Autodesk Inventor part; units mm, degrees
(part 2 of 2)
sketch "Sketch23" plane through (0, 0, 0) normal (0, 0, -1) x (-1, 0, 0)
  line L0 (124.7957, 172.4284) -> (124.7957, 166.0784) projected
  line L1 (124.7957, 166.0784) -> (73.9957, 166.0784) projected
  line L2 (73.9957, 166.0784) -> (73.9957, 172.4284) projected
  line L3 (73.9957, 172.4284) -> (23.1957, 172.4284) projected
  line L4 (23.1957, 172.4284) -> (23.1957, 166.0784) projected
  line L5 (23.1957, 166.0784) -> (-27.6043, 166.0784) projected
  line L6 (-27.6043, 166.0784) -> (-27.6043, 172.4284) projected
  line L7 (-27.6043, 172.4284) -> (-78.4043, 172.4284) projected
  line L8 (-78.4043, 172.4284) -> (-78.4043, 166.0784) projected
  line L9 (-78.4043, 166.0784) -> (-129.2043, 166.0784) projected
  line L10 (-129.2043, 166.0784) -> (-129.2043, 172.4284) projected
  line L11 (-129.2043, 172.4284) -> (-180.0043, 172.4284) projected
  line L12 (-180.0043, 172.4284) -> (-180.0043, 166.0784) projected
  line L13 (-180.0043, 166.0784) -> (-230.8043, 166.0784) projected
  line L14 (-230.8043, 166.0784) -> (-230.8043, 172.4284) projected
  line L15 (-230.8043, 172.4284) -> (-281.6043, 172.4284) projected
  line L16 (-281.6043, 172.4284) -> (-281.6043, 166.0784) projected
  line L17 (-281.6043, 166.0784) -> (-332.4043, 166.0784) projected
  line L18 (-332.4043, 166.0784) -> (-332.4043, 172.4284) projected
  line L19 (-332.4043, 172.4284) -> (-351.4543, 172.4284) projected
  line L20 (-351.4543, 172.4284) -> (-351.4543, 121.6284) projected
  line L21 (-351.4543, 121.6284) -> (-345.1043, 121.6284) projected
  line L22 (-345.1043, 121.6284) -> (-345.1043, 70.8284) projected
  line L23 (-345.1043, 70.8284) -> (-351.4543, 70.8284) projected
  line L24 (-351.4543, 70.8284) -> (-351.4543, 20.0284) projected
  line L25 (-351.4543, 20.0284) -> (-345.1043, 20.0284) projected
  line L26 (-345.1043, 20.0284) -> (-345.1043, -30.7716) projected
  line L27 (-345.1043, -30.7716) -> (-351.4543, -30.7716) projected
  line L28 (-351.4543, -30.7716) -> (-351.4543, -81.5716) projected
  line L29 (-351.4543, -81.5716) -> (-345.1043, -81.5716) projected
  line L30 (-345.1043, -81.5716) -> (-345.1043, -132.3716) projected
  line L31 (-345.1043, -132.3716) -> (-351.4543, -132.3716) projected
  line L32 (-351.4543, -132.3716) -> (-351.4543, -183.1716) projected
  line L33 (-351.4543, -183.1716) -> (-345.1043, -183.1716) projected
  line L34 (-345.1043, -183.1716) -> (-345.1043, -233.9716) projected
  line L35 (-345.1043, -233.9716) -> (-351.4543, -233.9716) projected
  line L36 (-351.4543, -233.9716) -> (-351.4543, -284.7716) projected
  line L37 (-351.4543, -284.7716) -> (-345.1043, -284.7716) projected
  line L38 (-345.1043, -284.7716) -> (-345.1043, -335.5716) projected
  line L39 (-345.1043, -335.5716) -> (-351.4543, -335.5716) projected
  line L40 (-351.4543, -335.5716) -> (-351.4543, -386.3716) projected
  line L41 (-351.4543, -386.3716) -> (-345.1043, -386.3716) projected
  line L42 (-345.1043, -386.3716) -> (-345.1043, -437.1716) projected
  line L43 (-345.1043, -437.1716) -> (-351.4543, -437.1716) projected
  line L44 (-351.4543, -437.1716) -> (-351.4543, -487.9716) projected
  line L45 (-351.4543, -487.9716) -> (-345.1043, -487.9716) projected
  line L46 (-345.1043, -487.9716) -> (-345.1043, -538.7716) projected
  line L47 (-345.1043, -538.7716) -> (-351.4543, -538.7716) projected
  line L48 (-351.4543, -538.7716) -> (-351.4543, -589.5716) projected
  line L49 (-351.4543, -589.5716) -> (-345.1043, -589.5716) projected
  line L50 (-345.1043, -589.5716) -> (-345.1043, -640.3716) projected
  line L51 (-345.1043, -640.3716) -> (-351.4543, -640.3716) projected
  line L52 (-351.4543, -640.3716) -> (-351.4543, -716.5716) projected
  line L53 (-351.4543, -716.5716) -> (-332.4043, -716.5716) projected
  line L54 (-332.4043, -716.5716) -> (-332.4043, -710.2216) projected
  line L55 (-332.4043, -710.2216) -> (-281.6043, -710.2216) projected
  line L56 (-281.6043, -710.2216) -> (-281.6043, -716.5716) projected
  line L57 (-281.6043, -716.5716) -> (-230.8043, -716.5716) projected
  line L58 (-230.8043, -716.5716) -> (-230.8043, -710.2216) projected
  line L59 (-230.8043, -710.2216) -> (-180.0043, -710.2216) projected
  line L60 (-180.0043, -710.2216) -> (-180.0043, -716.5716) projected
  line L61 (-180.0043, -716.5716) -> (-129.2043, -716.5716) projected
  line L62 (-129.2043, -716.5716) -> (-129.2043, -710.2216) projected
  line L63 (-129.2043, -710.2216) -> (-78.4043, -710.2216) projected
  line L64 (-78.4043, -710.2216) -> (-78.4043, -716.5716) projected
  line L65 (-78.4043, -716.5716) -> (-27.6043, -716.5716) projected
  line L66 (-27.6043, -716.5716) -> (-27.6043, -710.2216) projected
  line L67 (-27.6043, -710.2216) -> (23.1957, -710.2216) projected
  line L68 (23.1957, -710.2216) -> (23.1957, -716.5716) projected
  line L69 (23.1957, -716.5716) -> (73.9957, -716.5716) projected
  line L70 (73.9957, -716.5716) -> (73.9957, -710.2216) projected
  line L71 (73.9957, -710.2216) -> (124.7957, -710.2216) projected
  line L72 (124.7957, -710.2216) -> (124.7957, -716.5716) projected
  line L73 (124.7957, -716.5716) -> (143.8457, -716.5716) projected
  line L74 (143.8457, -716.5716) -> (143.8457, -640.3716) projected
  line L75 (143.8457, -640.3716) -> (137.4957, -640.3716) projected
  line L76 (137.4957, -640.3716) -> (137.4957, -589.5716) projected
  line L77 (137.4957, -589.5716) -> (143.8457, -589.5716) projected
  line L78 (143.8457, -589.5716) -> (143.8457, -538.7716) projected
  line L79 (143.8457, -538.7716) -> (137.4957, -538.7716) projected
  line L80 (137.4957, -538.7716) -> (137.4957, -487.9716) projected
  line L81 (137.4957, -487.9716) -> (143.8457, -487.9716) projected
  line L82 (143.8457, -487.9716) -> (143.8457, -437.1716) projected
  line L83 (143.8457, -437.1716) -> (137.4957, -437.1716) projected
  line L84 (137.4957, -437.1716) -> (137.4957, -386.3716) projected
  line L85 (137.4957, -386.3716) -> (143.8457, -386.3716) projected
  line L86 (143.8457, -386.3716) -> (143.8457, -335.5716) projected
  line L87 (143.8457, -335.5716) -> (137.4957, -335.5716) projected
  line L88 (137.4957, -335.5716) -> (137.4957, -284.7716) projected
  line L89 (137.4957, -284.7716) -> (143.8457, -284.7716) projected
  line L90 (143.8457, -284.7716) -> (143.8457, -233.9716) projected
  line L91 (143.8457, -233.9716) -> (137.4957, -233.9716) projected
  line L92 (137.4957, -233.9716) -> (137.4957, -183.1716) projected
  line L93 (137.4957, -183.1716) -> (143.8457, -183.1716) projected
  line L94 (143.8457, -183.1716) -> (143.8457, -132.3716) projected
  line L95 (143.8457, -132.3716) -> (137.4957, -132.3716) projected
  line L96 (137.4957, -132.3716) -> (137.4957, -81.5716) projected
  line L97 (137.4957, -81.5716) -> (143.8457, -81.5716) projected
  line L98 (143.8457, -81.5716) -> (143.8457, -30.7716) projected
  line L99 (143.8457, -30.7716) -> (137.4957, -30.7716) projected
  line L100 (137.4957, -30.7716) -> (137.4957, 20.0284) projected
  line L101 (137.4957, 20.0284) -> (143.8457, 20.0284) projected
  line L102 (143.8457, 20.0284) -> (143.8457, 70.8284) projected
  line L103 (143.8457, 70.8284) -> (137.4957, 70.8284) projected
  line L104 (137.4957, 70.8284) -> (137.4957, 121.6284) projected
  line L105 (137.4957, 121.6284) -> (143.8457, 121.6284) projected
  line L106 (143.8457, 121.6284) -> (143.8457, 172.4284) projected
  line L107 (143.8457, 172.4284) -> (124.7957, 172.4284) projected
  line L108 (-351.4543, 172.4284) -> (143.8457, 172.4284)
  line L109 (143.8457, 172.4284) -> (143.8457, -716.5716)
  line L110 (143.8457, -716.5716) -> (-351.4543, -716.5716)
  line L111 (-351.4543, -716.5716) -> (-351.4543, 172.4284)
  line L112 (124.7957, -699.4992) -> (-323.907, -699.4992)
  line L113 (-323.907, -699.4992) -> (-323.907, 137.5099)
  line L114 (-323.907, 137.5099) -> (124.7957, 137.5099)
  line L115 (124.7957, 137.5099) -> (124.7957, -699.4992)
  point P0 (0, 0)
  constraints: 16 end point, 4 parallel, 2 horizontal, 2 perpendicular
extrude "Extrusion23" add sketch "Sketch23" against normal blind 6.35 contours L107 L106 L105 L104 L103 L102 L101 L100 L99 L98 L97 L96 L95 L94 L93 L92 L91 L90 L89 L88 L87 L86 L85 L84 L83 L82 L81 L80 L79 L78 L77 L76 L75 L74 L73 L72 L71 L70 L69 L68 L67 L66 L65 L64 L63 L62 L61 L60 L59 L58 L57 L56 L55 L54 L53 L52 L51 L50 L49 L48 L47 L46 L45 L44 L43 L42 L41 L40 L39 L38 L37 L36 L35 L34 L33 L32 L31 L30 L29 L28 L27 L26 L25 L24 L23 L22 L21 L20 L19 L18 L17 L16 L15 L14 L13 L12 L11 L10 L9 L8 L7 L6 L5 L4 L3 L2 L1 L0 | L0 L1 L2 L108 | L109 L103 L104 L105 | L4 L5 L6 L108 | L109 L99 L100 L101 | L8 L9 L10 L108 | L109 L95 L96 L97 | L12 L13 L14 L108 | L109 L91 L92 L93 | L16 L17 L18 L108 | L109 L87 L88 L89 | L109 L83 L84 L85 | L109 L79 L80 L81 | L109 L75 L76 L77
sketch "Sketch24" plane through (0, 0, 0) normal (0, 0, -1) x (-1, 0, 0)
  line L0 (143.8457, 172.4284) -> (-351.4543, 172.4284) projected
  line L1 (-351.4543, 172.4284) -> (-351.4543, 121.6284) projected
  line L2 (-351.4543, 121.6284) -> (-345.1043, 121.6284) projected
  line L3 (-345.1043, 121.6284) -> (-345.1043, 70.8284) projected
  line L4 (-345.1043, 70.8284) -> (-351.4543, 70.8284) projected
  line L5 (-351.4543, 70.8284) -> (-351.4543, 20.0284) projected
  line L6 (-351.4543, 20.0284) -> (-345.1043, 20.0284) projected
  line L7 (-345.1043, 20.0284) -> (-345.1043, -30.7716) projected
  line L8 (-345.1043, -30.7716) -> (-351.4543, -30.7716) projected
  line L9 (-351.4543, -30.7716) -> (-351.4543, -81.5716) projected
  line L10 (-351.4543, -81.5716) -> (-345.1043, -81.5716) projected
  line L11 (-345.1043, -81.5716) -> (-345.1043, -132.3716) projected
  line L12 (-345.1043, -132.3716) -> (-351.4543, -132.3716) projected
  line L13 (-351.4543, -132.3716) -> (-351.4543, -183.1716) projected
  line L14 (-351.4543, -183.1716) -> (-345.1043, -183.1716) projected
  line L15 (-345.1043, -183.1716) -> (-345.1043, -233.9716) projected
  line L16 (-345.1043, -233.9716) -> (-351.4543, -233.9716) projected
  line L17 (-351.4543, -233.9716) -> (-351.4543, -284.7716) projected
  line L18 (-351.4543, -284.7716) -> (-345.1043, -284.7716) projected
  line L19 (-345.1043, -284.7716) -> (-345.1043, -335.5716) projected
  line L20 (-345.1043, -335.5716) -> (-351.4543, -335.5716) projected
  line L21 (-351.4543, -335.5716) -> (-351.4543, -386.3716) projected
  line L22 (-351.4543, -386.3716) -> (-345.1043, -386.3716) projected
  line L23 (-345.1043, -386.3716) -> (-345.1043, -437.1716) projected
  line L24 (-345.1043, -437.1716) -> (-351.4543, -437.1716) projected
  line L25 (-351.4543, -437.1716) -> (-351.4543, -487.9716) projected
  line L26 (-351.4543, -487.9716) -> (-345.1043, -487.9716) projected
  line L27 (-345.1043, -487.9716) -> (-345.1043, -538.7716) projected
  line L28 (-345.1043, -538.7716) -> (-351.4543, -538.7716) projected
  line L29 (-351.4543, -538.7716) -> (-351.4543, -589.5716) projected
  line L30 (-351.4543, -589.5716) -> (-345.1043, -589.5716) projected
  line L31 (-345.1043, -589.5716) -> (-345.1043, -640.3716) projected
  line L32 (-345.1043, -640.3716) -> (-351.4543, -640.3716) projected
  line L33 (-351.4543, -640.3716) -> (-351.4543, -716.5716) projected
  line L34 (-351.4543, -716.5716) -> (-332.4043, -716.5716) projected
  line L35 (-332.4043, -716.5716) -> (-332.4043, -710.2216) projected
  line L36 (-332.4043, -710.2216) -> (-281.6043, -710.2216) projected
  line L37 (-281.6043, -710.2216) -> (-281.6043, -716.5716) projected
  line L38 (-281.6043, -716.5716) -> (-230.8043, -716.5716) projected
  line L39 (-230.8043, -716.5716) -> (-230.8043, -710.2216) projected
  line L40 (-230.8043, -710.2216) -> (-180.0043, -710.2216) projected
  line L41 (-180.0043, -710.2216) -> (-180.0043, -716.5716) projected
  line L42 (-180.0043, -716.5716) -> (-129.2043, -716.5716) projected
  line L43 (-129.2043, -716.5716) -> (-129.2043, -710.2216) projected
  line L44 (-129.2043, -710.2216) -> (-78.4043, -710.2216) projected
  line L45 (-78.4043, -710.2216) -> (-78.4043, -716.5716) projected
  line L46 (-78.4043, -716.5716) -> (-27.6043, -716.5716) projected
  line L47 (-27.6043, -716.5716) -> (-27.6043, -710.2216) projected
  line L48 (-27.6043, -710.2216) -> (23.1957, -710.2216) projected
  line L49 (23.1957, -710.2216) -> (23.1957, -716.5716) projected
  line L50 (23.1957, -716.5716) -> (73.9957, -716.5716) projected
  line L51 (73.9957, -716.5716) -> (73.9957, -710.2216) projected
  line L52 (73.9957, -710.2216) -> (124.7957, -710.2216) projected
  line L53 (124.7957, -710.2216) -> (124.7957, -716.5716) projected
  line L54 (124.7957, -716.5716) -> (143.8457, -716.5716) projected
  line L55 (143.8457, -716.5716) -> (143.8457, 172.4284) projected
  line L56 (-351.4543, 121.6284) -> (-351.4543, -640.3716)
  line L57 (-332.4043, -716.5716) -> (124.7957, -716.5716)
  point P0 (0, 0)
  constraints: 4 end point, 1 parallel, 1 perpendicular
extrude "Extrusion24" add sketch "Sketch24" against normal blind 6.35 contours L2 L3 L4 L56 | L57 L51 L52 L53 | L6 L7 L8 L56 | L57 L47 L48 L49 | L10 L11 L12 L56 | L57 L43 L44 L45 | L14 L15 L16 L56 | L57 L39 L40 L41 | L18 L19 L20 L56 | L57 L35 L36 L37 | L22 L23 L24 L56 | L56 L30 L31 L32 | L26 L27 L28 L56
sketch "Sketch25" plane through (0, 0, 0) normal (0, 0, -1) x (-1, 0, 0)
  line L0 (143.8457, 172.4284) -> (-351.4543, 172.4284) projected
  line L1 (-351.4543, 172.4284) -> (-351.4543, -716.5716) projected
  line L2 (143.8457, -716.5716) -> (143.8457, 172.4284) projected
  line L3 (-351.4543, 172.4284) -> (-351.4543, 74.3844)
  line L4 (-351.4543, 74.3844) -> (143.8457, 74.3844)
  point P0 (0, 0)
  dimension "d150" = 98.044
  constraints: 4 end point, 2 point on line, 1 perpendicular
  measures "d150" distance of L0.end L3.end
extrude "Extrusion25" cut sketch "Sketch25" against normal blind 25.4
sketch "Sketch26" plane through (0, 0, 0) normal (0, 0, -1) x (-1, 0, 0)
  line L0 (143.8457, -716.5716) -> (143.8457, 74.3844) projected
  line L1 (-307.0043, -678.4716) -> (99.3957, -678.4716) projected
  line L2 (-351.4543, 74.3844) -> (-351.4543, 80.7344)
  line L3 (-351.4543, 80.7344) -> (143.8457, 80.7344)
  line L4 (143.8457, 80.7344) -> (143.8457, 42.6344)
  line L5 (143.8457, 42.6344) -> (-351.4543, 42.6344)
  line L6 (-351.4543, 42.6344) -> (-351.4543, 80.7344)
  point P0 (0, 0)
  dimension "d153" = 6.35
  dimension "d154" = 38.1
  constraints: 10 end point, 2 parallel, 2 perpendicular, 1 horizontal, 1 point on line
  measures "d153" distance of L2.start L2.end
  measures "d154" distance of L3.end L4.end
extrude "Extrusion26" add sketch "Sketch26" against normal blind 6.35
fillet "Fillet3" radius 6.35 2 edges at (-105.7457, 42.6344, 3.175) (313.3543, 42.6344, 3.175)
sketch "Sketch27" plane through (0, 0, 0) normal (0, 0, -1) x (-1, 0, 0)
  line L0 (-351.4543, 80.7344) -> (-351.4543, -716.5716) projected
  line L1 (143.8457, 80.7344) -> (-351.4543, 80.7344)
  line L2 (-351.4543, 80.7344) -> (-351.4543, 36.2844)
  line L3 (-351.4543, 36.2844) -> (143.8457, 36.2844)
  line L4 (143.8457, 36.2844) -> (143.8457, 80.7344)
  point P0 (0, 0)
  constraints: 8 end point, 2 parallel, 1 horizontal, 1 perpendicular, 1 point on line
extrude "Extrusion27" add sketch "Sketch27" against normal blind 6.35
sketch "Sketch28" plane through (0, 0, 0) normal (0, 0, -1) x (-1, 0, 0)
  line L0 (143.8457, -716.5716) -> (143.8457, 80.7344) projected
  line L1 (143.8457, 80.7344) -> (-351.4543, 80.7344) projected
  line L2 (-351.4543, 80.7344) -> (143.8457, 80.7344)
  line L3 (143.8457, 80.7344) -> (143.8457, 74.3844)
  line L4 (143.8457, 74.3844) -> (-351.4543, 74.3844)
  line L5 (-351.4543, 74.3844) -> (-351.4543, 80.7344)
  point P0 (0, 0)
  dimension "d160" = 6.35
  constraints: 8 end point, 2 parallel, 1 horizontal, 1 perpendicular, 1 point on line
  measures "d160" distance of L2.end L3.end
extrude "Extrusion28" cut sketch "Sketch28" against normal blind 6.35
fillet "Fillet4" radius 6.35 2 edges at (313.3543, 36.2844, 3.175) (-105.7457, 36.2844, 3.175)
body "Solid1"
